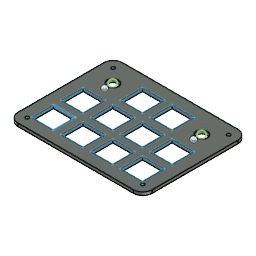
topplate,  done (Autodesk Fusion 360 design; units mm, degrees)
part number: 2026-03-29-14-58-47-218
Autodesk Fusion 360 part; units mm, degrees
sketch "Sketch1" plane through (0, 0, 0) normal (0, 0, 1) x (1, 0, 0)
  line L0 (0, 0) -> (86.2, 0)
  line L1 (86.2, 0) -> (86.2, -67.2)
  line L2 (86.2, -67.2) -> (0, -67.2)
  line L3 (0, -67.2) -> (0, 0)
  dimension "d1" = 86.2
  dimension "d2" = 67.2
  constraint horizontal L0
  constraint vertical L1
  constraint horizontal L2
  constraint vertical L3
  constraint coincident L0.start L3.end
  measures "d1" distance of L0.start L0.end
  measures "d2" distance of L0.start L2.end
extrude "Extrude1" add sketch "Sketch1" along normal blind 2
fillet "Fillet1" radius 6 4 edges at (0, -67.2, 1) (86.2, -67.2, 1) (86.2, 0, 1) (0, 0, 1)
sketch "Sketch2" plane through (0, 0, 2) normal (0, 0, 1) x (-1, 0, 0)
  arc A0 (-6, 0) -> (0, 6) centre (-6, 6) ccw
  line L0 (0, 6) -> (0, 61.2)
  arc A1 (0, 61.2) -> (-6, 67.2) centre (-6, 61.2) ccw
  line L1 (-6, 67.2) -> (-80.2, 67.2)
  arc A2 (-80.2, 67.2) -> (-86.2, 61.2) centre (-80.2, 61.2) ccw
  line L2 (-86.2, 61.2) -> (-86.2, 6)
  arc A3 (-86.2, 6) -> (-80.2, 0) centre (-80.2, 6) ccw
  line L3 (-80.2, 0) -> (-6, 0)
  circle A4 centre (-80.2, 61.2) radius 1.1
  circle A5 centre (-6, 61.2) radius 1.1
  circle A6 centre (-6, 6) radius 1.1
  circle A7 centre (-80.2, 6) radius 1.1
  dimension "d7" = 2.2
  dimension "d8" = 2.2
  dimension "d9" = 2.2
  dimension "d10" = 2.2
  dimension "d11" = 6
  dimension "d12" = 6
  dimension "d13" = 6
  dimension "d14" = 6
  dimension "d15" = 6
  dimension "d16" = 6
  dimension "d17" = 6
  dimension "d18" = 6
  measures "d7" diameter of A4
  measures "d8" diameter of A5
  measures "d9" diameter of A6
  measures "d10" diameter of A7
  measures "d11" distance of L2 A2.centre
  measures "d12" distance of L1 A2.centre
  measures "d13" distance of L0 A1.centre
  measures "d14" distance of L1 A1.centre
  measures "d15" distance of L3 A0.centre
  measures "d16" distance of L0 A0.centre
  measures "d17" distance of L3 A3.centre
  measures "d18" distance of L2 A3.centre
hole "Hole1" at (80.2, -61.2, 2) at (6, -61.2, 2) at (6, -6, 2) at (80.2, -6, 2) direction (0, 0, -1) diameter 2.2 depth 2.2 tip angle 118
sketch "Sketch4" plane through (0, 0, 2) normal (0, 0, 1) x (-1, 0, 0)
  circle A0 centre (-6, 6) radius 1.1
  circle A1 centre (-80.2, 61.2) radius 1.1
  circle A2 centre (-6, 61.2) radius 1.1
  circle A3 centre (-80.2, 6) radius 1.1
  arc A4 (-6, 0) -> (0, 6) centre (-6, 6) ccw
  line L0 (0, 6) -> (0, 61.2)
  arc A5 (0, 61.2) -> (-6, 67.2) centre (-6, 61.2) ccw
  line L1 (-6, 67.2) -> (-80.2, 67.2)
  arc A6 (-80.2, 67.2) -> (-86.2, 61.2) centre (-80.2, 61.2) ccw
  line L2 (-86.2, 61.2) -> (-86.2, 6)
  arc A7 (-86.2, 6) -> (-80.2, 0) centre (-80.2, 6) ccw
  line L3 (-80.2, 0) -> (-6, 0)
  line L4 (-21.4, 59.8) -> (-21.4, 45.8)
  line L5 (-21.4, 45.8) -> (-7.4, 45.8)
  line L6 (-26.45, 45.8) -> (-26.45, 59.8)
  line L7 (-40.45, 45.8) -> (-26.45, 45.8)
  line L8 (-40.45, 59.8) -> (-40.45, 45.8)
  line L9 (-26.45, 59.8) -> (-40.45, 59.8)
  line L10 (-45.5, 45.8) -> (-45.5, 59.8)
  line L11 (-59.5, 45.8) -> (-45.5, 45.8)
  line L12 (-59.5, 59.8) -> (-59.5, 45.8)
  line L13 (-45.5, 59.8) -> (-59.5, 59.8)
  line L14 (-64.55, 45.8) -> (-64.55, 59.8)
  line L15 (-78.55, 45.8) -> (-64.55, 45.8)
  line L16 (-78.55, 59.8) -> (-78.55, 45.8)
  line L17 (-64.55, 59.8) -> (-78.55, 59.8)
  line L18 (-7.4, 26.75) -> (-7.4, 40.75)
  line L19 (-21.4, 26.75) -> (-7.4, 26.75)
  line L20 (-21.4, 40.75) -> (-21.4, 26.75)
  line L21 (-7.4, 40.75) -> (-21.4, 40.75)
  line L22 (-26.45, 26.75) -> (-26.45, 40.75)
  line L23 (-40.45, 26.75) -> (-26.45, 26.75)
  line L24 (-40.45, 40.75) -> (-40.45, 26.75)
  line L25 (-26.45, 40.75) -> (-40.45, 40.75)
  line L26 (-45.5, 26.75) -> (-45.5, 40.75)
  line L27 (-59.5, 26.75) -> (-45.5, 26.75)
  line L28 (-59.5, 40.75) -> (-59.5, 26.75)
  line L29 (-45.5, 40.75) -> (-59.5, 40.75)
  line L30 (-64.55, 26.75) -> (-64.55, 40.75)
  line L31 (-78.55, 26.75) -> (-64.55, 26.75)
  line L32 (-78.55, 40.75) -> (-78.55, 26.75)
  line L33 (-64.55, 40.75) -> (-78.55, 40.75)
  line L34 (-26.45, 7.7) -> (-26.45, 21.7)
  line L35 (-40.45, 7.7) -> (-26.45, 7.7)
  line L36 (-40.45, 21.7) -> (-40.45, 7.7)
  line L37 (-26.45, 21.7) -> (-40.45, 21.7)
  line L38 (-45.5, 7.7) -> (-45.5, 21.7)
  line L39 (-59.5, 7.7) -> (-45.5, 7.7)
  line L40 (-59.5, 21.7) -> (-59.5, 7.7)
  line L41 (-45.5, 21.7) -> (-59.5, 21.7)
  line L42 (-7.4, 45.8) -> (-21.4, 45.8)
  line L43 (-21.4, 45.8) -> (-21.4, 59.8)
  line L44 (-21.4, 59.8) -> (-7.4, 59.8)
  line L45 (-7.4, 59.8) -> (-7.4, 45.8)
  circle A8 centre (-14.4, 14.7) radius 3.5
  circle A9 centre (-71.55, 14.7) radius 3.5
  circle A10 centre (-14.4, 19.9) radius 1
  circle A11 centre (-71.55, 19.9) radius 1
  dimension "d41" = 7
  dimension "d42" = 7
  dimension "d43" = 2
  dimension "d44" = 5.2
  dimension "d45" = 2
  dimension "d46" = 5.2
  constraint vertical L4
  constraint horizontal L5
  constraint horizontal L42
  constraint vertical L43
  constraint horizontal L44
  constraint vertical L45
  measures "d41" diameter of A8
  measures "d42" diameter of A9
  measures "d43" diameter of A10
  measures "d44" distance of A8.centre A10.centre
  measures "d45" diameter of A11
  measures "d46" distance of A9.centre A11.centre
extrude "Extrude2" cut sketch "Sketch4" against normal blind 2 contours L4 L5 L42 L43 L44 L45 | L6 L7 L8 L9 | L10 L11 L12 L13 | L14 L15 L16 L17 | L18 L19 L20 L21 | L22 L23 L24 L25 | L26 L27 L28 L29 | L30 L31 L32 L33 | L34 L35 L36 L37 | L38 L39 L40 L41
extrude "Extrude3" cut sketch "Sketch4" against normal blind 2 contours A8 | A9 | A10 | A11
sketch "Sketch5" plane through (0, 0, 2) normal (0, 0, 1) x (-1, 0, 0)
